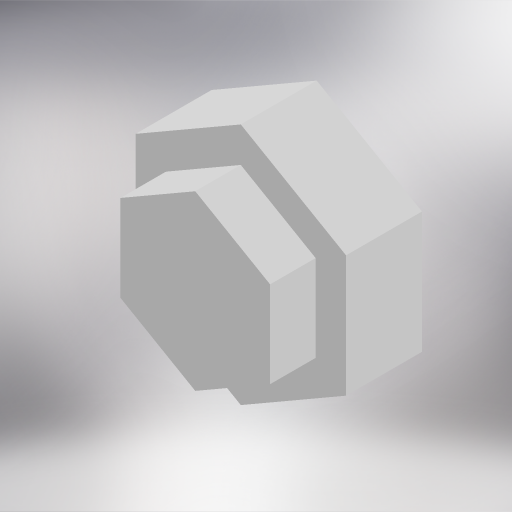
# Autodesk Inventor part: white_part1
Saved by Autodesk Inventor 2024 (Build 280153000, 153)
## iProperties
Created: 2023-10-25
Part Number: white_part1
Material: Generic
Document SubType Name: Modeling
Designer: SSAFY
Density: 1 g/cm^3
Appearance: Default
Author: SSAFY
Autodesk Inventor part; units mm, degrees
ref_plane "YZ Plane" through (0, 0, 0) normal (1, 0, 0) x (0, 1, 0)
ref_plane "XZ Plane" through (0, 0, 0) normal (0, 1, 0) x (-1, 0, 0)
ref_plane "XY Plane" through (0, 0, 0) normal (0, 0, 1) x (1, 0, 0)
sketch "Sketch1" plane through (0, 0, 0) normal (0, 0, 1) x (1, 0, 0)
  line L0 (0, 8) -> (6.9282, 4)
  line L1 (6.9282, 4) -> (6.9282, -4)
  line L2 (6.9282, -4) -> (0, -8)
  line L3 (0, -8) -> (-6.9282, -4)
  line L4 (-6.9282, -4) -> (-6.9282, 4)
  line L5 (-6.9282, 4) -> (0, 8)
  point P0 (0, 0)
  point P1 (0, 0)
  dimension "d0" = 8
  constraints: 12 end point, 1 coincident, 13 other
  measures "d0" distance of L3.end L4.end
extrude "Extrusion1" add sketch "Sketch1" along normal blind 5
sketch "Sketch2" plane through (0, 0, 5) normal (0, 0, 1) x (1, 0, 0)
  line L0 (-6.9282, 4) -> (-6.9282, -4) projected
  line L1 (-6.9282, -4) -> (0, -8) projected
  line L2 (0, -8) -> (6.9282, -4) projected
  line L3 (6.9282, -4) -> (6.9282, 4) projected
  line L4 (6.9282, 4) -> (0, 8) projected
  line L5 (0, 8) -> (-6.9282, 4) projected
  line L6 (-4.9282, 2.8453) -> (-4.9282, -2.8453)
  line L7 (-4.9282, -2.8453) -> (0, -5.6906)
  line L8 (0, -5.6906) -> (4.9282, -2.8453)
  line L9 (4.9282, -2.8453) -> (4.9282, 2.8453)
  line L10 (4.9282, 2.8453) -> (0, 5.6906)
  line L11 (0, 5.6906) -> (-4.9282, 2.8453)
  point P0 (0, 0)
  dimension "d3" = 2
  constraints: 12 end point, 5 other
  measures "d3" distance between parallel lines of L11 L5
extrude "Extrusion2" add sketch "Sketch2" along normal blind 3 contours L11 L10 L9 L8 L7 L6
sketch "Sketch3" plane through (0, 0, 0) normal (0, 0, -1) x (-1, 0, 0)
  circle A0 centre (0, 0) radius 2.5
  dimension "d6" = 5
  constraints: 1 centre point, 1 coincident
  measures "d6" diameter of A0
extrude "Extrusion3" cut sketch "Sketch3" against normal blind 5
chamfer "Chamfer1" distance 1 angle 45 1 edges at (2.5, 0, 0)
body "Solid1"
